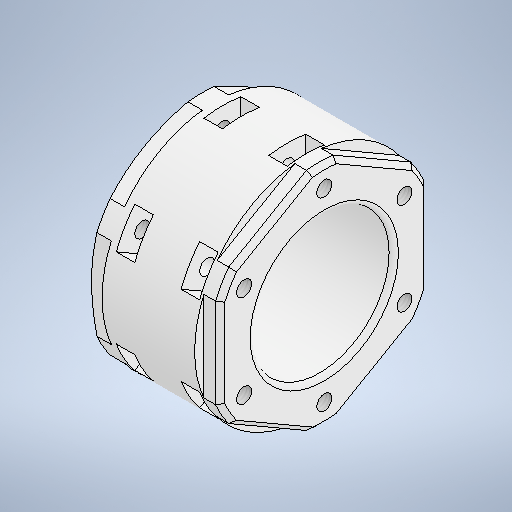
# Autodesk Inventor part: joint4_axis3
Saved by Autodesk Inventor 2025.3 (Build 293356030, 356C)
## iProperties
Created: 2025-10-28
Part Number: joint4_axis3
Material: PLA filament
Document SubType Name: Modeling
Designer: MSI
Density: 1.2 g/cm^3
Appearance: 일반
Mass: 34.174 g
Surface Area: 124.256 cm^2
Volume: 28.4784 cm^3
Author: MSI
Autodesk Inventor part; units mm, degrees
ref_plane "YZ Plane" through (0, 0, 0) normal (1, 0, 0) x (0, 1, 0)
ref_plane "XZ Plane" through (0, 0, 0) normal (0, 1, 0) x (-1, 0, 0)
ref_plane "XY Plane" through (0, 0, 0) normal (0, 0, 1) x (1, 0, 0)
sketch "스케치1" plane through (0, 0, 0) normal (0, 0, 1) x (1, 0, 0)
  line L0 (0, 0) -> (29.5, 0)
  line L1 (29.5, 0) -> (29.5, 24.5)
  line L2 (29.5, 24.5) -> (0, 24.5)
  line L3 (0, 24.5) -> (0, 0)
  line L4 (6, 0) -> (7.5, 0)
  dimension "d3" = 49
  dimension "d12" = 29.5
  constraints: 10 end point, 2 horizontal, 2 parallel, 1 perpendicular, 1 point on line
  measures "d3" diameter of L2 L0
  measures "d12" distance of L1.end L2.end
revolve "회전1" add sketch "스케치1" angle 360 about axis through (0, 0, 0) along (1, 0, 0)
sketch "스케치3" plane through (29.5, 0, 0) normal (1, 0, 0) x (0, 0, -1)
  circle A0 centre (0, 0) radius 24.5 projected
  constraints: 1 coincident
hole "구멍2" at (29.5, 0, 0) direction (-1, 0, 0) diameter 30 end through all
chamfer "모따기1" distance 5 angle 30 1 edges at (0, -24.5, 0) measured on face at (0, -24, 0)
sketch "스케치4" plane through (0, 0, 0) normal (-1, 0, 0) x (0, 0, 1)
  circle A0 centre (0, 0) radius 24.5 projected
  line L0 (0, 25.9808) -> (22.5, 12.9904)
  line L1 (22.5, 12.9904) -> (22.5, -12.9904)
  line L2 (22.5, -12.9904) -> (0, -25.9808)
  line L3 (0, -25.9808) -> (-22.5, -12.9904)
  line L4 (-22.5, -12.9904) -> (-22.5, 12.9904)
  line L5 (-22.5, 12.9904) -> (0, 25.9808)
  point P0 (2.8536, 24.3333)
  point P1 (19.6464, 14.6379)
  point P2 (22.5, 9.6954)
  point P3 (22.5, -9.6954)
  point P4 (19.6464, -14.6379)
  point P5 (2.8536, -24.3333)
  point P6 (-2.8536, -24.3333)
  point P7 (-19.6464, -14.6379)
  point P8 (-22.5, -9.6954)
  point P9 (-22.5, 9.6954)
  point P10 (-19.6464, 14.6379)
  point P11 (-2.8536, 24.3333)
  dimension "d27" = 45
  constraints: 12 end point, 1 coincident, 1 vertical alignment, 13 other
  measures "d27" distance between parallel lines of L1 L4
extrude "돌출1" cut sketch "스케치4" against normal blind 6 contours A0 L1 | L0 A0 | A0 L2 | L5 A0 | A0 L3 | L4 A0
sketch "스케치8" plane through (0, 0, 0) normal (-1, 0, 0) x (0, 0, 1)
  line L0 (0, 0) -> (0, 20)
  dimension "d45" = 20
  constraints: 2 end point, 1 vertical
  measures "d45" distance of L0.start L0.end
hole "구멍4" at (0, 20, 0) direction (1, 0, 0) diameter 3.242 depth 19 tip angle 118 thread size "M4x0.7" class "6H" standard "ISO Metric profile"
pattern_circular "원형 패턴2" count 6 over 360 about axis through (-45.8143, 0, 0) along (1, 0, 0) of "구멍4"
sketch "스케치6" plane through (29.5, 0, 0) normal (1, 0, 0) x (0, 0, -1)
  line L0 (0, 25.9808) -> (22.5, 12.9904)
  line L1 (22.5, 12.9904) -> (22.5, -12.9904)
  line L2 (22.5, -12.9904) -> (0, -25.9808)
  line L3 (0, -25.9808) -> (-22.5, -12.9904)
  line L4 (-22.5, -12.9904) -> (-22.5, 12.9904)
  line L5 (-22.5, 12.9904) -> (0, 25.9808)
  circle A0 centre (0, 0) radius 24.5 projected
  point P0 (2.8536, -24.3333)
  point P1 (19.6464, -14.6379)
  point P2 (-19.6464, -14.6379)
  point P3 (-2.8536, -24.3333)
  point P4 (22.5, 9.6954)
  point P5 (22.5, -9.6954)
  point P6 (-22.5, 9.6954)
  point P7 (-22.5, -9.6954)
  point P8 (19.6464, 14.6379)
  point P9 (2.8536, 24.3333)
  point P10 (-2.8536, 24.3333)
  point P11 (-19.6464, 14.6379)
  dimension "d28" = 45
  constraints: 12 end point, 1 coincident, 1 vertical alignment, 13 other
  measures "d28" distance between parallel lines of L1 L4
extrude "돌출2" cut sketch "스케치6" against normal blind 3.5 contours L0 A0 L5 | A0 L0 | L5 A0 | L0 L1 A0 | A0 L4 L5 | A0 L1 | L4 A0 | L1 L2 A0 | A0 L3 L4 | A0 L2 | L3 A0 | L2 L3 A0
sketch "스케치9" plane through (29.5, -9.6954, -22.5) normal (1, 0, 0) x (0, 0, -1)
  line L0 (-22.5, 9.6954) -> (-22.5, 29.6954)
  dimension "d56" = 20
  constraints: 2 end point, 1 vertical
  measures "d56" distance of L0.start L0.end
hole "구멍5" at (29.5, 20, 0) direction (-1, 0, 0) diameter 3.242 depth 11.8 tip angle 118 thread size "M4x0.7" class "6H" standard "ISO Metric profile"
pattern_circular "원형 패턴3" count 6 over 360 about axis through (-45.8143, 0, 0) along (1, 0, 0) of "구멍5"
chamfer "모따기3" distance 1 angle 45 13 edges at (29.5, 0, 22.5) (29.5, 12.25, 21.2176) (29.5, 19.4856, 11.25) (29.5, 24.4583, -1.4292) (29.5, 24.4583, 1.4292) (29.5, 19.4856, -11.25) (29.5, 12.25, -21.2176) (29.5, -12.25, -21.2176) (29.5, 0, -22.5) (29.5, -19.4856, -11.25) (29.5, -24.5, 0) (29.5, -19.4856, 11.25) (29.5, -12.25, 21.2176)
fillet "모깎기2" radius 1 1 edges at (29.5, 0, 15)
ref_plane "작업 평면2" through (25.5, -9.4868, -21.5) normal (1, 0, 0) x (0, 0, -1)
sketch "스케치10" plane through (25.5, -9.4868, -21.5) normal (1, 0, 0) x (0, 0, -1)
  circle A0 centre (-21.5, 29.4868) radius 1.621 projected
  line L0 (-21.5, 34.1056) -> (-17.5, 31.7962)
  line L1 (-17.5, 31.7962) -> (-17.5, 27.1774)
  line L2 (-17.5, 27.1774) -> (-21.5, 24.868)
  line L3 (-21.5, 24.868) -> (-25.5, 27.1774)
  line L4 (-25.5, 27.1774) -> (-25.5, 31.7962)
  line L5 (-25.5, 31.7962) -> (-21.5, 34.1056)
  line L6 (-25.5, 31.7962) -> (-25.5, 40.476)
  line L7 (-25.5, 40.476) -> (-17.5, 40.476)
  line L8 (-17.5, 40.476) -> (-17.5, 31.7962)
  point P0 (-21.5, 9.4868)
  dimension "d78" = 8
  constraints: 18 end point, 2 perpendicular, 1 coincident, 1 point on line, 1 vertical, 1 vertical alignment, 13 other
  measures "d78" distance of L6.end L7.end
extrude "돌출3" cut sketch "스케치10" against normal blind 4 contours A0 | L5 L6 L7 L8 L0 | L0 L1 L2 L3 L4 L5
ref_plane "작업 평면3" through (7.5, 20, 0) normal (-1, 0, 0) x (0, 0, 1)
sketch "스케치11" plane through (7.5, 20, 0) normal (-1, 0, 0) x (0, 0, 1)
  circle A0 centre (0, 0) radius 1.621 projected
  line L0 (0, -4.6188) -> (4, -2.3094) projected
  line L1 (0, -4.6188) -> (-4, -2.3094)
  line L2 (-4, -2.3094) -> (-4, 2.3094)
  line L3 (-4, 2.3094) -> (0, 4.6188)
  line L4 (0, 4.6188) -> (4, 2.3094)
  line L5 (4, 2.3094) -> (4, -2.3094)
  line L6 (4, -2.3094) -> (0, -4.6188)
  line L7 (-4, 2.3094) -> (-4, 6.7155)
  line L8 (-4, 6.7155) -> (4, 6.7155)
  line L9 (4, 6.7155) -> (4, 2.3094)
  arc A1 (4, 4.1713) -> (-4, 4.1713) centre (0, -20) ccw projected
  point P0 (4, -2.3094)
  constraints: 18 end point, 1 coincident, 1 collinear, 1 perpendicular, 1 point on line, 1 vertical, 13 other
extrude "돌출4" cut sketch "스케치11" against normal blind 4 contours A0 | L1 L2 L3 A1 L4 L5 L0 | L4 A1 L9 | L7 A1 L3 | A1 L3 L4 | L4 L3 A1 L7 L8 L9
pattern_circular "원형 패턴4" count 6 over 360 about axis through (-45.8143, 0, 0) along (1, 0, 0) of "돌출4", "돌출3"
equation "\"d13\" = joint4_axis3_d1"
equation "\"joint4_belt_centor\" = 157.367"
equation "\"joint4_axis2_L\" = 58.803"
equation "\"joint4_axis2_b1\" = 35"
equation "\"joint4_axis2_d\" = 19"
equation "\"joint4_miter_m\" = 2"
equation "\"joint4_miter_a\" = 20deg"
equation "\"joint4_miter_z\" = 79"
equation "\"joint4_miter_b\" = 6.90139"
equation "\"joint4_axis3_L\" = 23.5"
equation "\"joint4_axis3_d1\" = 30"
equation "\"joint3_belt_centor\" = 157.367"
equation "\"joint3_axis2_L\" = 16"
equation "\"joint3_axis2_d\" = 19"
equation "\"joint3_planetary_m\" = 1.5"
equation "\"joint3_planetary_a\" = 20deg"
equation "\"joint3_planetary_np\" = 4"
equation "\"joint3_sun_z\" = 18"
equation "\"joint3_sun_b\" = 17"
equation "\"joint3_planet_z\" = 36"
equation "\"joint3_planet_b\" = 17"
equation "\"joint3_ring_b\" = 9"
equation "\"joint3_axis3_d\" = 29"
equation "\"joint3_miter_m\" = 5.5"
equation "\"joint3_miter_a\" = 20deg"
equation "\"joint3_miter_z\" = 28"
equation "\"joint3_miter_b\" = 13.65957"
equation "\"joint3_axis4_L\" = 23.5"
